Autodesk Fusion 360 part; units mm, degrees
note: some values were not read from the file. Set by a fixed rule: which sketch regions a step uses.
(part 13 of 20)
  spline S72 degree 5 poles (-2.755, -30.8773) (-2.7539, -30.8749) (-2.7515, -30.87) (-2.748, -30.8627) (-2.7434, -30.853) (-2.7376, -30.8408) (-2.7319, -30.8287) (-2.7262, -30.8165) (-2.7205, -30.8044) (-2.7149, -30.7924) (-2.7092, -30.7803) (-2.7036, -30.7683) (-2.6981, -30.7563) (-2.6925, -30.7443) (-2.687, -30.7323) (-2.6815, -30.7204) (-2.6761, -30.7085) (-2.6707, -30.6966) (-2.6653, -30.6847) (-2.6599, -30.6728) (-2.6545, -30.661) (-2.6492, -30.6492) (-2.6439, -30.6374) (-2.6387, -30.6256) (-2.6335, -30.6139) (-2.6283, -30.6022) (-2.6231, -30.5905) (-2.6179, -30.5788) (-2.6128, -30.5672) (-2.6077, -30.5555) (-2.6027, -30.5439) (-2.5977, -30.5324) (-2.5927, -30.5208) (-2.5877, -30.5093) (-2.5827, -30.4978) (-2.5778, -30.4863) (-2.5729, -30.4749) (-2.5681, -30.4634) (-2.5632, -30.452) (-2.5584, -30.4407) (-2.5537, -30.4293) (-2.5489, -30.418) (-2.5442, -30.4067) (-2.5395, -30.3954) (-2.5348, -30.3841) (-2.5302, -30.3729) (-2.5256, -30.3617) (-2.521, -30.3506) (-2.5165, -30.3394) (-2.5119, -30.3283) (-2.5074, -30.3172) (-2.503, -30.3061) (-2.4985, -30.2951) (-2.4941, -30.2841) (-2.4897, -30.2731) (-2.4854, -30.2621) (-2.481, -30.2512) (-2.4767, -30.2403) (-2.4725, -30.2294) (-2.4682, -30.2186) (-2.464, -30.2078) (-2.4598, -30.197) (-2.4557, -30.1862) (-2.4515, -30.1755) (-2.4474, -30.1648) (-2.4433, -30.1541) (-2.4393, -30.1435) (-2.4353, -30.1329) (-2.4313, -30.1223) (-2.4273, -30.1118) (-2.4234, -30.1012) (-2.4194, -30.0907) (-2.4156, -30.0803) (-2.4117, -30.0699) (-2.4079, -30.0595) (-2.4041, -30.0491) (-2.4003, -30.0388) (-2.3965, -30.0284) (-2.3928, -30.0182) (-2.3891, -30.0079) (-2.3855, -29.9977) (-2.3818, -29.9875) (-2.3782, -29.9774) (-2.3746, -29.9673) (-2.3711, -29.9572) (-2.3675, -29.9471) (-2.364, -29.9371) (-2.3606, -29.9271) (-2.3571, -29.9172) (-2.3537, -29.9073) (-2.3503, -29.8974) (-2.3469, -29.8875) (-2.3436, -29.8777) (-2.3403, -29.868) (-2.337, -29.8582) (-2.3337, -29.8485) (-2.3305, -29.8388) (-2.3273, -29.8292) (-2.3241, -29.8196) (-2.321, -29.81) (-2.3178, -29.8005) (-2.3147, -29.791) (-2.3117, -29.7815) (-2.3086, -29.7721) (-2.3056, -29.7627) (-2.3026, -29.7534) (-2.2996, -29.7441) (-2.2967, -29.7348) (-2.2938, -29.7255) (-2.2909, -29.7163) (-2.288, -29.7072) (-2.2852, -29.6981) (-2.2824, -29.689) (-2.2796, -29.6799) (-2.2769, -29.6709) (-2.2741, -29.6619) (-2.2714, -29.653) (-2.2688, -29.6441) (-2.2661, -29.6353) (-2.2635, -29.6265) (-2.2609, -29.6177) (-2.2583, -29.609) (-2.2558, -29.6003) (-2.2533, -29.5917) (-2.2508, -29.583) (-2.2483, -29.5745) (-2.2458, -29.566) (-2.2434, -29.5575) (-2.241, -29.5491) (-2.2387, -29.5407) (-2.2363, -29.5323) (-2.234, -29.524) (-2.2317, -29.5158) (-2.2295, -29.5075) (-2.2272, -29.4994) (-2.225, -29.4912) (-2.2228, -29.4832) (-2.2207, -29.4751) (-2.2185, -29.4671) (-2.2164, -29.4592) (-2.2143, -29.4513) (-2.2123, -29.4434) (-2.2102, -29.4356) (-2.2082, -29.4279) (-2.2062, -29.4202) (-2.2043, -29.4125) (-2.2023, -29.4049) (-2.2004, -29.3973) (-2.1985, -29.3898) (-2.1967, -29.3823) (-2.1948, -29.3749) (-2.193, -29.3675) (-2.1912, -29.3602) (-2.1895, -29.3529) (-2.1877, -29.3457) (-2.186, -29.3386) (-2.1843, -29.3314) (-2.1827, -29.3244) (-2.181, -29.3174) (-2.1794, -29.3104) (-2.1778, -29.3035) (-2.1762, -29.2967) (-2.1747, -29.2899) (-2.1731, -29.2831) (-2.1716, -29.2764) (-2.1702, -29.2698) (-2.1687, -29.2632) (-2.1673, -29.2567) (-2.1659, -29.2502) (-2.1645, -29.2438) (-2.1631, -29.2374) (-2.1618, -29.2311) (-2.1605, -29.2249) (-2.1592, -29.2187) (-2.1579, -29.2126) (-2.1567, -29.2065) (-2.1554, -29.2005) (-2.1542, -29.1946) (-2.153, -29.1887) (-2.1519, -29.1829) (-2.1507, -29.1771) (-2.1496, -29.1714) (-2.1485, -29.1658) (-2.1475, -29.1602) (-2.1464, -29.1547) (-2.1454, -29.1493) (-2.1444, -29.1439) (-2.1434, -29.1386) (-2.1424, -29.1334) (-2.1415, -29.1282) (-2.1406, -29.1231) (-2.1397, -29.118) (-2.1388, -29.1131) (-2.138, -29.1081) (-2.1371, -29.1033) (-2.1363, -29.0985) (-2.1355, -29.0938) (-2.1347, -29.0892) (-2.134, -29.0847) (-2.1332, -29.0802) (-2.1325, -29.0758) (-2.1318, -29.0714) (-2.1312, -29.0672) (-2.1305, -29.063) (-2.1299, -29.0589) (-2.1292, -29.0549) (-2.1286, -29.0509) (-2.1281, -29.047) (-2.1275, -29.0432) (-2.127, -29.0395) (-2.1264, -29.0359) (-2.1259, -29.0323) (-2.1254, -29.0289) (-2.125, -29.0255) (-2.1245, -29.0222) (-2.1241, -29.0189) (-2.1237, -29.0158) (-2.1233, -29.0128) (-2.1229, -29.0098) (-2.1225, -29.0069) (-2.1222, -29.0041) (-2.1219, -29.0015) (-2.1215, -28.9989) (-2.1212, -28.9963) (-2.121, -28.9939) (-2.1207, -28.9916) (-2.1204, -28.9894) (-2.1202, -28.9873) (-2.12, -28.9852) (-2.1198, -28.9833) (-2.1196, -28.9815) (-2.1194, -28.9798) (-2.1192, -28.9781) (-2.1191, -28.9766) (-2.1189, -28.9752) (-2.1188, -28.9739) (-2.1187, -28.9727) (-2.1186, -28.9716) (-2.1185, -28.9706) (-2.1184, -28.9698) (-2.1184, -28.969) (-2.1183, -28.9685) (-2.1183, -28.9682) (-2.1183, -28.968) (-2.1183, -28.9679) knots -1 -1 -1 -1 -1 -1 -0.99583333 -0.99166667 -0.9875 -0.98333333 -0.97916667 -0.975 -0.97083333 -0.96666667 -0.9625 -0.95833333 -0.95416667 -0.95 -0.94583333 -0.94166667 -0.9375 -0.93333333 -0.92916667 -0.925 -0.92083333 -0.91666667 -0.9125 -0.90833333 -0.90416667 -0.9 -0.89583333 -0.89166667 -0.8875 -0.88333333 -0.87916667 -0.875 -0.87083333 -0.86666667 -0.8625 -0.85833333 -0.85416667 -0.85 -0.84583333 -0.84166667 -0.8375 -0.83333333 -0.82916667 -0.825 -0.82083333 -0.81666667 -0.8125 -0.80833333 -0.80416667 -0.8 -0.79583333 -0.79166667 -0.7875 -0.78333333 -0.77916667 -0.775 -0.77083333 -0.76666667 -0.7625 -0.75833333 -0.75416667 -0.75 -0.74583333 -0.74166667 -0.7375 -0.73333333 -0.72916667 -0.725 -0.72083333 -0.71666667 -0.7125 -0.70833333 -0.70416667 -0.7 -0.69583333 -0.69166667 -0.6875 -0.68333333 -0.67916667 -0.675 -0.67083333 -0.66666667 -0.6625 -0.65833333 -0.65416667 -0.65 -0.64583333 -0.64166667 -0.6375 -0.63333333 -0.62916667 -0.625 -0.62083333 -0.61666667 -0.6125 -0.60833333 -0.60416667 -0.6 -0.59583333 -0.59166667 -0.5875 -0.58333333 -0.57916667 -0.575 -0.57083333 -0.56666667 -0.5625 -0.55833333 -0.55416667 -0.55 -0.54583333 -0.54166667 -0.5375 -0.53333333 -0.52916667 -0.525 -0.52083333 -0.51666667 -0.5125 -0.50833333 -0.50416667 -0.5 -0.49583333 -0.49166667 -0.4875 -0.48333333 -0.47916667 -0.475 -0.47083333 -0.46666667 -0.4625 -0.45833333 -0.45416667 -0.45 -0.44583333 -0.44166667 -0.4375 -0.43333333 -0.42916667 -0.425 -0.42083333 -0.41666667 -0.4125 -0.40833333 -0.40416667 -0.4 -0.39583333 -0.39166667 -0.3875 -0.38333333 -0.37916667 -0.375 -0.37083333 -0.36666667 -0.3625 -0.35833333 -0.35416667 -0.35 -0.34583333 -0.34166667 -0.3375 -0.33333333 -0.32916667 -0.325 -0.32083333 -0.31666667 -0.3125 -0.30833333 -0.30416667 -0.3 -0.29583333 -0.29166667 -0.2875 -0.28333333 -0.27916667 -0.275 -0.27083333 -0.26666667 -0.2625 -0.25833333 -0.25416667 -0.25 -0.24583333 -0.24166667 -0.2375 -0.23333333 -0.22916667 -0.225 -0.22083333 -0.21666667 -0.2125 -0.20833333 -0.20416667 -0.2 -0.19583333 -0.19166667 -0.1875 -0.18333333 -0.17916667 -0.175 -0.17083333 -0.16666667 -0.1625 -0.15833333 -0.15416667 -0.15 -0.14583333 -0.14166667 -0.1375 -0.13333333 -0.12916667 -0.125 -0.12083333 -0.11666667 -0.1125 -0.10833333 -0.10416667 -0.1 -0.09583333 -0.09166667 -0.0875 -0.08333333 -0.07916667 -0.075 -0.07083333 -0.06666667 -0.0625 -0.05833333 -0.05416667 -0.05 -0.04583333 -0.04166667 -0.0375 -0.03333333 -0.02916667 -0.025 -0.02083333 -0.01666667 -0.0125 -0.00833333 -0.00416667 0 0 0 0 0 0
  spline S73 degree 5 poles (26.8955, 10.9662) (26.8956, 10.9662) (26.8958, 10.9663) (26.8961, 10.9664) (26.8966, 10.9666) (26.8973, 10.9669) (26.8981, 10.9672) (26.899, 10.9676) (26.9, 10.9681) (26.9011, 10.9685) (26.9023, 10.9691) (26.9036, 10.9696) (26.905, 10.9702) (26.9065, 10.9709) (26.908, 10.9716) (26.9097, 10.9724) (26.9115, 10.9731) (26.9134, 10.974) (26.9153, 10.9749) (26.9173, 10.9758) (26.9195, 10.9768) (26.9217, 10.9778) (26.924, 10.9788) (26.9263, 10.9799) (26.9288, 10.9811) (26.9313, 10.9823) (26.9339, 10.9835) (26.9366, 10.9848) (26.9394, 10.9861) (26.9423, 10.9875) (26.9452, 10.9889) (26.9482, 10.9903) (26.9513, 10.9918) (26.9544, 10.9934) (26.9577, 10.9949) (26.961, 10.9966) (26.9643, 10.9982) (26.9678, 10.9999) (26.9713, 11.0017) (26.9748, 11.0035) (26.9785, 11.0053) (26.9822, 11.0072) (26.986, 11.0091) (26.9898, 11.0111) (26.9937, 11.0131) (26.9977, 11.0151) (27.0017, 11.0172) (27.0058, 11.0193) (27.01, 11.0215) (27.0142, 11.0237) (27.0185, 11.0259) (27.0228, 11.0282) (27.0272, 11.0306) (27.0317, 11.0329) (27.0362, 11.0353) (27.0408, 11.0378) (27.0454, 11.0403) (27.0501, 11.0428) (27.0549, 11.0454) (27.0597, 11.048) (27.0645, 11.0507) (27.0694, 11.0534) (27.0744, 11.0561) (27.0794, 11.0589) (27.0845, 11.0617) (27.0896, 11.0646) (27.0948, 11.0675) (27.1, 11.0704) (27.1053, 11.0734) (27.1106, 11.0764) (27.116, 11.0795) (27.1214, 11.0826) (27.1269, 11.0857) (27.1324, 11.0889) (27.138, 11.0921) (27.1436, 11.0954) (27.1493, 11.0987) (27.155, 11.102) (27.1608, 11.1054) (27.1666, 11.1088) (27.1725, 11.1123) (27.1784, 11.1158) (27.1843, 11.1193) (27.1903, 11.1229) (27.1963, 11.1265) (27.2024, 11.1301) (27.2085, 11.1338) (27.2147, 11.1376) (27.2209, 11.1413) (27.2271, 11.1451) (27.2334, 11.149) (27.2397, 11.1529) (27.2461, 11.1568) (27.2525, 11.1608) (27.259, 11.1648) (27.2654, 11.1688) (27.272, 11.1729) (27.2785, 11.177) (27.2851, 11.1812) (27.2918, 11.1854) (27.2985, 11.1896) (27.3052, 11.1939) (27.3119, 11.1982) (27.3187, 11.2025) (27.3256, 11.2069) (27.3324, 11.2113) (27.3393, 11.2158) (27.3463, 11.2203) (27.3533, 11.2248) (27.3603, 11.2294) (27.3673, 11.234) (27.3744, 11.2387) (27.3815, 11.2434) (27.3887, 11.2481) (27.3958, 11.2529) (27.4031, 11.2577) (27.4103, 11.2625) (27.4176, 11.2674) (27.4249, 11.2723) (27.4323, 11.2773) (27.4396, 11.2823) (27.447, 11.2873) (27.4545, 11.2924) (27.462, 11.2975) (27.4695, 11.3026) (27.477, 11.3078) (27.4846, 11.313) (27.4922, 11.3183) (27.4998, 11.3235) (27.5074, 11.3289) (27.5151, 11.3342) (27.5228, 11.3396) (27.5306, 11.3451) (27.5384, 11.3506) (27.5462, 11.3561) (27.554, 11.3616) (27.5618, 11.3672) (27.5697, 11.3728) (27.5776, 11.3785) (27.5856, 11.3842) (27.5936, 11.3899) (27.6015, 11.3957) (27.6096, 11.4015) (27.6176, 11.4074) (27.6257, 11.4132) (27.6338, 11.4192) (27.6419, 11.4251) (27.6501, 11.4311) (27.6582, 11.4371) (27.6665, 11.4432) (27.6747, 11.4493) (27.6829, 11.4554) (27.6912, 11.4616) (27.6995, 11.4678) (27.7078, 11.4741) (27.7162, 11.4803) (27.7246, 11.4867) (27.733, 11.493) (27.7414, 11.4994) (27.7498, 11.5058) (27.7583, 11.5123) (27.7668, 11.5188) (27.7753, 11.5253) (27.7838, 11.5319) (27.7924, 11.5385) (27.801, 11.5452) (27.8096, 11.5518) (27.8182, 11.5585) (27.8268, 11.5653) (27.8355, 11.5721) (27.8442, 11.5789) (27.8529, 11.5858) (27.8616, 11.5927) (27.8704, 11.5996) (27.8791, 11.6065) (27.8879, 11.6135) (27.8967, 11.6206) (27.9055, 11.6276) (27.9144, 11.6348) (27.9233, 11.6419) (27.9322, 11.6491) (27.9411, 11.6563) (27.95, 11.6635) (27.9589, 11.6708) (27.9679, 11.6781) (27.9769, 11.6855) (27.9859, 11.6929) (27.9949, 11.7003) (28.0039, 11.7078) (28.013, 11.7153) (28.0221, 11.7228) (28.0312, 11.7303) (28.0403, 11.7379) (28.0494, 11.7456) (28.0585, 11.7532) (28.0677, 11.7609) (28.0769, 11.7687) (28.0861, 11.7765) (28.0953, 11.7843) (28.1045, 11.7921) (28.1137, 11.8) (28.123, 11.8079) (28.1323, 11.8158) (28.1416, 11.8238) (28.1509, 11.8318) (28.1602, 11.8399) (28.1695, 11.848) (28.1789, 11.8561) (28.1882, 11.8643) (28.1976, 11.8724) (28.207, 11.8807) (28.2164, 11.8889) (28.2259, 11.8972) (28.2353, 11.9055) (28.2447, 11.9139) (28.2542, 11.9223) (28.2637, 11.9307) (28.2732, 11.9392) (28.2827, 11.9477) (28.2922, 11.9562) (28.3018, 11.9648) (28.3113, 11.9734) (28.3209, 11.982) (28.3305, 11.9907) (28.34, 11.9994) (28.3496, 12.0081) (28.3593, 12.0169) (28.3689, 12.0257) (28.3785, 12.0345) (28.3882, 12.0434) (28.3978, 12.0523) (28.4075, 12.0613) (28.4172, 12.0702) (28.4269, 12.0792) (28.4366, 12.0883) (28.4464, 12.0973) (28.4561, 12.1065) (28.4658, 12.1156) (28.4756, 12.1248) (28.4854, 12.134) (28.4951, 12.1432) (28.503, 12.1506) (28.5089, 12.1562) (28.5128, 12.16) (28.5147, 12.1618) knots 0 0 0 0 0 0 0.00416667 0.00833333 0.0125 0.01666667 0.02083333 0.025 0.02916667 0.03333333 0.0375 0.04166667 0.04583333 0.05 0.05416667 0.05833333 0.0625 0.06666667 0.07083333 0.075 0.07916667 0.08333333 0.0875 0.09166667 0.09583333 0.1 0.10416667 0.10833333 0.1125 0.11666667 0.12083333 0.125 0.12916667 0.13333333 0.1375 0.14166667 0.14583333 0.15 0.15416667 0.15833333 0.1625 0.16666667 0.17083333 0.175 0.17916667 0.18333333 0.1875 0.19166667 0.19583333 0.2 0.20416667 0.20833333 0.2125 0.21666667 0.22083333 0.225 0.22916667 0.23333333 0.2375 0.24166667 0.24583333 0.25 0.25416667 0.25833333 0.2625 0.26666667 0.27083333 0.275 0.27916667 0.28333333 0.2875 0.29166667 0.29583333 0.3 0.30416667 0.30833333 0.3125 0.31666667 0.32083333 0.325 0.32916667 0.33333333 0.3375 0.34166667 0.34583333 0.35 0.35416667 0.35833333 0.3625 0.36666667 0.37083333 0.375 0.37916667 0.38333333 0.3875 0.39166667 0.39583333 0.4 0.40416667 0.40833333 0.4125 0.41666667 0.42083333 0.425 0.42916667 0.43333333 0.4375 0.44166667 0.44583333 0.45 0.45416667 0.45833333 0.4625 0.46666667 0.47083333 0.475 0.47916667 0.48333333 0.4875 0.49166667 0.49583333 0.5 0.50416667 0.50833333 0.5125 0.51666667 0.52083333 0.525 0.52916667 0.53333333 0.5375 0.54166667 0.54583333 0.55 0.55416667 0.55833333 0.5625 0.56666667 0.57083333 0.575 0.57916667 0.58333333 0.5875 0.59166667 0.59583333 0.6 0.60416667 0.60833333 0.6125 0.61666667 0.62083333 0.625 0.62916667 0.63333333 0.6375 0.64166667 0.64583333 0.65 0.65416667 0.65833333 0.6625 0.66666667 0.67083333 0.675 0.67916667 0.68333333 0.6875 0.69166667 0.69583333 0.7 0.70416667 0.70833333 0.7125 0.71666667 0.72083333 0.725 0.72916667 0.73333333 0.7375 0.74166667 0.74583333 0.75 0.75416667 0.75833333 0.7625 0.76666667 0.77083333 0.775 0.77916667 0.78333333 0.7875 0.79166667 0.79583333 0.8 0.80416667 0.80833333 0.8125 0.81666667 0.82083333 0.825 0.82916667 0.83333333 0.8375 0.84166667 0.84583333 0.85 0.85416667 0.85833333 0.8625 0.86666667 0.87083333 0.875 0.87916667 0.88333333 0.8875 0.89166667 0.89583333 0.9 0.90416667 0.90833333 0.9125 0.91666667 0.92083333 0.925 0.92916667 0.93333333 0.9375 0.94166667 0.94583333 0.95 0.95416667 0.95833333 0.9625 0.96666667 0.97083333 0.975 0.97916667 0.98333333 0.9875 0.99166667 0.99583333 1 1 1 1 1 1
  line L156 (-20.11, 20.9575) -> (-20.1094, 20.9569)
  spline S74 degree 5 poles (-0.9213, -29.0307) (-0.9213, -29.0307) (-0.9213, -29.0309) (-0.9213, -29.0313) (-0.9213, -29.0318) (-0.9213, -29.0325) (-0.9213, -29.0334) (-0.9214, -29.0344) (-0.9214, -29.0355) (-0.9214, -29.0367) (-0.9214, -29.038) (-0.9214, -29.0394) (-0.9214, -29.0409) (-0.9214, -29.0425) (-0.9214, -29.0443) (-0.9214, -29.0461) (-0.9214, -29.0481) (-0.9214, -29.0501) (-0.9214, -29.0522) (-0.9214, -29.0545) (-0.9214, -29.0568) (-0.9213, -29.0592) (-0.9213, -29.0618) (-0.9212, -29.0644) (-0.9212, -29.0671) (-0.9211, -29.0699) (-0.9211, -29.0728) (-0.921, -29.0758) (-0.9209, -29.0788) (-0.9208, -29.082) (-0.9208, -29.0852) (-0.9206, -29.0886) (-0.9205, -29.092) (-0.9204, -29.0955) (-0.9203, -29.0991) (-0.9201, -29.1028) (-0.92, -29.1065) (-0.9198, -29.1103) (-0.9197, -29.1143) (-0.9195, -29.1183) (-0.9193, -29.1223) (-0.9191, -29.1265) (-0.9189, -29.1307) (-0.9186, -29.135) (-0.9184, -29.1394) (-0.9182, -29.1439) (-0.9179, -29.1484) (-0.9176, -29.153) (-0.9173, -29.1577) (-0.917, -29.1624) (-0.9167, -29.1673) (-0.9164, -29.1722) (-0.9161, -29.1771) (-0.9157, -29.1822) (-0.9153, -29.1873) (-0.915, -29.1925) (-0.9146, -29.1977) (-0.9141, -29.203) (-0.9137, -29.2084) (-0.9133, -29.2139) (-0.9128, -29.2194) (-0.9124, -29.225) (-0.9119, -29.2306) (-0.9114, -29.2363) (-0.9109, -29.2421) (-0.9103, -29.248) (-0.9098, -29.2539) (-0.9092, -29.2599) (-0.9087, -29.2659) (-0.9081, -29.272) (-0.9075, -29.2781) (-0.9068, -29.2844) (-0.9062, -29.2906) (-0.9055, -29.297) (-0.9049, -29.3034) (-0.9042, -29.3099) (-0.9035, -29.3164) (-0.9027, -29.323) (-0.902, -29.3296) (-0.9012, -29.3363) (-0.9005, -29.343) (-0.8997, -29.3498) (-0.8989, -29.3567) (-0.898, -29.3636) (-0.8972, -29.3706) (-0.8963, -29.3777) (-0.8954, -29.3847) (-0.8945, -29.3919) (-0.8936, -29.3991) (-0.8927, -29.4063) (-0.8917, -29.4137) (-0.8907, -29.421) (-0.8897, -29.4284) (-0.8887, -29.4359) (-0.8877, -29.4434) (-0.8866, -29.451) (-0.8856, -29.4586) (-0.8845, -29.4663) (-0.8834, -29.474) (-0.8822, -29.4818) (-0.8811, -29.4896) (-0.8799, -29.4975) (-0.8787, -29.5054) (-0.8775, -29.5134) (-0.8763, -29.5214) (-0.875, -29.5295) (-0.8738, -29.5376) (-0.8725, -29.5458) (-0.8712, -29.554) (-0.8698, -29.5623) (-0.8685, -29.5706) (-0.8671, -29.5789) (-0.8657, -29.5873) (-0.8643, -29.5958) (-0.8629, -29.6043) (-0.8614, -29.6128) (-0.86, -29.6214) (-0.8585, -29.6301) (-0.8569, -29.6388) (-0.8554, -29.6475) (-0.8538, -29.6563) (-0.8523, -29.6651) (-0.8507, -29.6739) (-0.849, -29.6828) (-0.8474, -29.6918) (-0.8457, -29.7008) (-0.844, -29.7098) (-0.8423, -29.7189) (-0.8406, -29.728) (-0.8388, -29.7372) (-0.8371, -29.7464) (-0.8353, -29.7556) (-0.8334, -29.7649) (-0.8316, -29.7742) (-0.8297, -29.7836) (-0.8279, -29.793) (-0.8259, -29.8025) (-0.824, -29.812) (-0.8221, -29.8215) (-0.8201, -29.8311) (-0.8181, -29.8407) (-0.8161, -29.8503) (-0.814, -29.86) (-0.812, -29.8697) (-0.8099, -29.8795) (-0.8078, -29.8893) (-0.8056, -29.8992) (-0.8035, -29.909) (-0.8013, -29.919) (-0.7991, -29.9289) (-0.7969, -29.9389) (-0.7946, -29.949) (-0.7923, -29.959) (-0.79, -29.9691) (-0.7877, -29.9793) (-0.7854, -29.9895) (-0.783, -29.9997) (-0.7806, -30.0099) (-0.7782, -30.0202) (-0.7758, -30.0306) (-0.7733, -30.0409) (-0.7708, -30.0513) (-0.7683, -30.0618) (-0.7658, -30.0722) (-0.7632, -30.0827) (-0.7606, -30.0933) (-0.758, -30.1038) (-0.7554, -30.1145) (-0.7528, -30.1251) (-0.7501, -30.1358) (-0.7474, -30.1465) (-0.7447, -30.1572) (-0.7419, -30.168) (-0.7391, -30.1788) (-0.7364, -30.1897) (-0.7335, -30.2005) (-0.7307, -30.2114) (-0.7278, -30.2224) (-0.7249, -30.2334) (-0.722, -30.2444) (-0.7191, -30.2554) (-0.7161, -30.2665) (-0.7131, -30.2776) (-0.7101, -30.2887) (-0.7071, -30.2999) (-0.704, -30.3111) (-0.7009, -30.3223) (-0.6978, -30.3336) (-0.6947, -30.3448) (-0.6915, -30.3562) (-0.6883, -30.3675) (-0.6851, -30.3789) (-0.6819, -30.3903) (-0.6786, -30.4017) (-0.6753, -30.4132) (-0.672, -30.4247) (-0.6687, -30.4362) (-0.6653, -30.4478) (-0.6619, -30.4594) (-0.6585, -30.471) (-0.6551, -30.4827) (-0.6516, -30.4943) (-0.6481, -30.506) (-0.6446, -30.5178) (-0.6411, -30.5295) (-0.6375, -30.5413) (-0.6339, -30.5531) (-0.6303, -30.565) (-0.6267, -30.5769) (-0.623, -30.5888) (-0.6193, -30.6007) (-0.6156, -30.6126) (-0.6118, -30.6246) (-0.6081, -30.6366) (-0.6043, -30.6487) (-0.6005, -30.6607) (-0.5966, -30.6728) (-0.5927, -30.685) (-0.5889, -30.6971) (-0.5849, -30.7093) (-0.581, -30.7215) (-0.577, -30.7337) (-0.573, -30.7459) (-0.569, -30.7582) (-0.5649, -30.7705) (-0.5609, -30.7828) (-0.5568, -30.7952) (-0.5526, -30.8076) (-0.5485, -30.82) (-0.5443, -30.8324) (-0.5401, -30.8448) (-0.5359, -30.8573) (-0.5316, -30.8698) (-0.5273, -30.8823) (-0.523, -30.8949) (-0.5187, -30.9075) (-0.5143, -30.9201) (-0.5099, -30.9327) (-0.5055, -30.9453) (-0.5011, -30.958) (-0.4966, -30.9707) (-0.493, -30.9809) (-0.4903, -30.9885) (-0.4885, -30.9936) (-0.4876, -30.9962) knots 0 0 0 0 0 0 0.00416667 0.00833333 0.0125 0.01666667 0.02083333 0.025 0.02916667 0.03333333 0.0375 0.04166667 0.04583333 0.05 0.05416667 0.05833333 0.0625 0.06666667 0.07083333 0.075 0.07916667 0.08333333 0.0875 0.09166667 0.09583333 0.1 0.10416667 0.10833333 0.1125 0.11666667 0.12083333 0.125 0.12916667 0.13333333 0.1375 0.14166667 0.14583333 0.15 0.15416667 0.15833333 0.1625 0.16666667 0.17083333 0.175 0.17916667 0.18333333 0.1875 0.19166667 0.19583333 0.2 0.20416667 0.20833333 0.2125 0.21666667 0.22083333 0.225 0.22916667 0.23333333 0.2375 0.24166667 0.24583333 0.25 0.25416667 0.25833333 0.2625 0.26666667 0.27083333 0.275 0.27916667 0.28333333 0.2875 0.29166667 0.29583333 0.3 0.30416667 0.30833333 0.3125 0.31666667 0.32083333 0.325 0.32916667 0.33333333 0.3375 0.34166667 0.34583333 0.35 0.35416667 0.35833333 0.3625 0.36666667 0.37083333 0.375 0.37916667 0.38333333 0.3875 0.39166667 0.39583333 0.4 0.40416667 0.40833333 0.4125 0.41666667 0.42083333 0.425 0.42916667 0.43333333 0.4375 0.44166667 0.44583333 0.45 0.45416667 0.45833333 0.4625 0.46666667 0.47083333 0.475 0.47916667 0.48333333 0.4875 0.49166667 0.49583333 0.5 0.50416667 0.50833333 0.5125 0.51666667 0.52083333 0.525 0.52916667 0.53333333 0.5375 0.54166667 0.54583333 0.55 0.55416667 0.55833333 0.5625 0.56666667 0.57083333 0.575 0.57916667 0.58333333 0.5875 0.59166667 0.59583333 0.6 0.60416667 0.60833333 0.6125 0.61666667 0.62083333 0.625 0.62916667 0.63333333 0.6375 0.64166667 0.64583333 0.65 0.65416667 0.65833333 0.6625 0.66666667 0.67083333 0.675 0.67916667 0.68333333 0.6875 0.69166667 0.69583333 0.7 0.70416667 0.70833333 0.7125 0.71666667 0.72083333 0.725 0.72916667 0.73333333 0.7375 0.74166667 0.74583333 0.75 0.75416667 0.75833333 0.7625 0.76666667 0.77083333 0.775 0.77916667 0.78333333 0.7875 0.79166667 0.79583333 0.8 0.80416667 0.80833333 0.8125 0.81666667 0.82083333 0.825 0.82916667 0.83333333 0.8375 0.84166667 0.84583333 0.85 0.85416667 0.85833333 0.8625 0.86666667 0.87083333 0.875 0.87916667 0.88333333 0.8875 0.89166667 0.89583333 0.9 0.90416667 0.90833333 0.9125 0.91666667 0.92083333 0.925 0.92916667 0.93333333 0.9375 0.94166667 0.94583333 0.95 0.95416667 0.95833333 0.9625 0.96666667 0.97083333 0.975 0.97916667 0.98333333 0.9875 0.99166667 0.99583333 1 1 1 1 1 1
  spline S75 degree 5 poles (-13.7175, 25.6019) (-13.7175, 25.602) (-13.7176, 25.6022) (-13.7178, 25.6025) (-13.718, 25.6029) (-13.7184, 25.6036) (-13.7188, 25.6043) (-13.7193, 25.6052) (-13.7198, 25.6061) (-13.7204, 25.6072) (-13.721, 25.6083) (-13.7217, 25.6096) (-13.7225, 25.6109) (-13.7233, 25.6123) (-13.7242, 25.6138) (-13.7251, 25.6154) (-13.7261, 25.6171) (-13.7271, 25.6188) (-13.7282, 25.6207) (-13.7293, 25.6226) (-13.7305, 25.6246) (-13.7317, 25.6267) (-13.733, 25.6289) (-13.7344, 25.6311) (-13.7358, 25.6334) (-13.7372, 25.6358) (-13.7387, 25.6383) (-13.7403, 25.6409) (-13.7419, 25.6435) (-13.7435, 25.6462) (-13.7452, 25.6489) (-13.747, 25.6518) (-13.7488, 25.6547) (-13.7506, 25.6577) (-13.7526, 25.6607) (-13.7545, 25.6638) (-13.7565, 25.667) (-13.7586, 25.6702) (-13.7607, 25.6735) (-13.7628, 25.6769) (-13.765, 25.6803) (-13.7673, 25.6838) (-13.7696, 25.6874) (-13.7719, 25.691) (-13.7743, 25.6947) (-13.7768, 25.6984) (-13.7793, 25.7022) (-13.7818, 25.706) (-13.7844, 25.71) (-13.787, 25.7139) (-13.7897, 25.718) (-13.7925, 25.722) (-13.7952, 25.7262) (-13.7981, 25.7304) (-13.8009, 25.7346) (-13.8039, 25.7389) (-13.8068, 25.7432) (-13.8098, 25.7476) (-13.8129, 25.7521) (-13.816, 25.7566) (-13.8192, 25.7612) (-13.8224, 25.7658) (-13.8256, 25.7704) (-13.8289, 25.7751) (-13.8322, 25.7799) (-13.8356, 25.7847) (-13.839, 25.7895) (-13.8425, 25.7944) (-13.846, 25.7993) (-13.8496, 25.8043) (-13.8532, 25.8093) (-13.8568, 25.8144) (-13.8605, 25.8195) (-13.8643, 25.8247) (-13.8681, 25.8299) (-13.8719, 25.8352) (-13.8758, 25.8405) (-13.8797, 25.8458) (-13.8836, 25.8512) (-13.8876, 25.8566) (-13.8917, 25.8621) (-13.8958, 25.8676) (-13.8999, 25.8731) (-13.9041, 25.8787) (-13.9083, 25.8843) (-13.9126, 25.89) (-13.9169, 25.8957) (-13.9213, 25.9014) (-13.9257, 25.9072) (-13.9301, 25.913) (-13.9346, 25.9188) (-13.9391, 25.9247) (-13.9437, 25.9306) (-13.9483, 25.9366) (-13.9529, 25.9426) (-13.9576, 25.9486) (-13.9624, 25.9547) (-13.9672, 25.9608) (-13.972, 25.9669) (-13.9769, 25.9731) (-13.9818, 25.9793) (-13.9867, 25.9855) (-13.9917, 25.9918) (-13.9967, 25.9981) (-14.0018, 26.0044) (-14.0069, 26.0108) (-14.0121, 26.0172) (-14.0173, 26.0236) (-14.0225, 26.0301) (-14.0278, 26.0366) (-14.0332, 26.0431) (-14.0385, 26.0497) (-14.0439, 26.0563) (-14.0494, 26.0629) (-14.0549, 26.0695) (-14.0604, 26.0762) (-14.066, 26.0829) (-14.0716, 26.0896) (-14.0772, 26.0964) (-14.0829, 26.1032) (-14.0887, 26.11) (-14.0945, 26.1168) (-14.1003, 26.1237) (-14.1061, 26.1306) (-14.112, 26.1375) (-14.118, 26.1445) (-14.1239, 26.1515) (-14.13, 26.1585) (-14.136, 26.1655) (-14.1421, 26.1726) (-14.1483, 26.1796) (-14.1544, 26.1868) (-14.1607, 26.1939) (-14.1669, 26.201) (-14.1732, 26.2082) (-14.1796, 26.2154) (-14.1859, 26.2227) (-14.1924, 26.2299) (-14.1988, 26.2372) (-14.2053, 26.2445) (-14.2119, 26.2518) (-14.2184, 26.2592) (-14.225, 26.2665) (-14.2317, 26.2739) (-14.2384, 26.2813) (-14.2451, 26.2888) (-14.2519, 26.2962) (-14.2587, 26.3037) (-14.2656, 26.3112) (-14.2724, 26.3188) (-14.2794, 26.3263) (-14.2863, 26.3339) (-14.2933, 26.3414) (-14.3004, 26.3491) (-14.3075, 26.3567) (-14.3146, 26.3643) (-14.3217, 26.372) (-14.3289, 26.3797) (-14.3362, 26.3874) (-14.3435, 26.3951) (-14.3508, 26.4029) (-14.3581, 26.4106) (-14.3655, 26.4184) (-14.3729, 26.4262) (-14.3804, 26.434) (-14.3879, 26.4419) (-14.3954, 26.4497) (-14.403, 26.4576) (-14.4106, 26.4655) (-14.4183, 26.4734) (-14.426, 26.4813) (-14.4337, 26.4893) (-14.4415, 26.4972) (-14.4493, 26.5052) (-14.4571, 26.5132) (-14.465, 26.5212) (-14.4729, 26.5292) (-14.4809, 26.5373) (-14.4889, 26.5453) (-14.4969, 26.5534) (-14.505, 26.5615) (-14.5131, 26.5696) (-14.5212, 26.5777) (-14.5294, 26.5858) (-14.5376, 26.594) (-14.5459, 26.6022) (-14.5541, 26.6103) (-14.5625, 26.6185) (-14.5708, 26.6267) (-14.5792, 26.635) (-14.5877, 26.6432) (-14.5961, 26.6514) (-14.6046, 26.6597) (-14.6132, 26.668) (-14.6218, 26.6763) (-14.6304, 26.6846) (-14.639, 26.6929) (-14.6477, 26.7012) (-14.6565, 26.7096) (-14.6652, 26.7179) (-14.674, 26.7263) (-14.6829, 26.7347) (-14.6917, 26.7431) (-14.7006, 26.7515) (-14.7096, 26.7599) (-14.7186, 26.7683) (-14.7276, 26.7767) (-14.7366, 26.7852) (-14.7457, 26.7937) (-14.7549, 26.8021) (-14.764, 26.8106) (-14.7732, 26.8191) (-14.7824, 26.8276) (-14.7917, 26.8361) (-14.801, 26.8447) (-14.8104, 26.8532) (-14.8197, 26.8618) (-14.8291, 26.8703) (-14.8386, 26.8789) (-14.8481, 26.8875) (-14.8576, 26.8961) (-14.8671, 26.9047) (-14.8767, 26.9133) (-14.8863, 26.9219) (-14.896, 26.9305) (-14.9057, 26.9392) (-14.9154, 26.9478) (-14.9252, 26.9565) (-14.935, 26.9651) (-14.9448, 26.9738) (-14.9547, 26.9825) (-14.9646, 26.9912) (-14.9745, 26.9999) (-14.9845, 27.0086) (-14.9945, 27.0173) (-15.0045, 27.026) (-15.0146, 27.0347) (-15.0247, 27.0435) (-15.0349, 27.0522) (-15.045, 27.061) (-15.0553, 27.0697) (-15.0635, 27.0767) (-15.0696, 27.082) (-15.0737, 27.0855) (-15.0758, 27.0873) knots 0 0 0 0 0 0 0.00416667 0.00833333 0.0125 0.01666667 0.02083333 0.025 0.02916667 0.03333333 0.0375 0.04166667 0.04583333 0.05 0.05416667 0.05833333 0.0625 0.06666667 0.07083333 0.075 0.07916667 0.08333333 0.0875 0.09166667 0.09583333 0.1 0.10416667 0.10833333 0.1125 0.11666667 0.12083333 0.125 0.12916667 0.13333333 0.1375 0.14166667 0.14583333 0.15 0.15416667 0.15833333 0.1625 0.16666667 0.17083333 0.175 0.17916667 0.18333333 0.1875 0.19166667 0.19583333 0.2 0.20416667 0.20833333 0.2125 0.21666667 0.22083333 0.225 0.22916667 0.23333333 0.2375 0.24166667 0.24583333 0.25 0.25416667 0.25833333 0.2625 0.26666667 0.27083333 0.275 0.27916667 0.28333333 0.2875 0.29166667 0.29583333 0.3 0.30416667 0.30833333 0.3125 0.31666667 0.32083333 0.325 0.32916667 0.33333333 0.3375 0.34166667 0.34583333 0.35 0.35416667 0.35833333 0.3625 0.36666667 0.37083333 0.375 0.37916667 0.38333333 0.3875 0.39166667 0.39583333 0.4 0.40416667 0.40833333 0.4125 0.41666667 0.42083333 0.425 0.42916667 0.43333333 0.4375 0.44166667 0.44583333 0.45 0.45416667 0.45833333 0.4625 0.46666667 0.47083333 0.475 0.47916667 0.48333333 0.4875 0.49166667 0.49583333 0.5 0.50416667 0.50833333 0.5125 0.51666667 0.52083333 0.525 0.52916667 0.53333333 0.5375 0.54166667 0.54583333 0.55 0.55416667 0.55833333 0.5625 0.56666667 0.57083333 0.575 0.57916667 0.58333333 0.5875 0.59166667 0.59583333 0.6 0.60416667 0.60833333 0.6125 0.61666667 0.62083333 0.625 0.62916667 0.63333333 0.6375 0.64166667 0.64583333 0.65 0.65416667 0.65833333 0.6625 0.66666667 0.67083333 0.675 0.67916667 0.68333333 0.6875 0.69166667 0.69583333 0.7 0.70416667 0.70833333 0.7125 0.71666667 0.72083333 0.725 0.72916667 0.73333333 0.7375 0.74166667 0.74583333 0.75 0.75416667 0.75833333 0.7625 0.76666667 0.77083333 0.775 0.77916667 0.78333333 0.7875 0.79166667 0.79583333 0.8 0.80416667 0.80833333 0.8125 0.81666667 0.82083333 0.825 0.82916667 0.83333333 0.8375 0.84166667 0.84583333 0.85 0.85416667 0.85833333 0.8625 0.86666667 0.87083333 0.875 0.87916667 0.88333333 0.8875 0.89166667 0.89583333 0.9 0.90416667 0.90833333 0.9125 0.91666667 0.92083333 0.925 0.92916667 0.93333333 0.9375 0.94166667 0.94583333 0.95 0.95416667 0.95833333 0.9625 0.96666667 0.97083333 0.975 0.97916667 0.98333333 0.9875 0.99166667 0.99583333 1 1 1 1 1 1
  arc A76 (-17.8246, 25.363) -> (-18.6136, 24.7898) centre (0, 0) ccw
  line L157 (-9.8469, 27.3243) -> (-9.7471, 27.0473)
  arc A77 (-12.5209, 25.8803) -> (-13.578, 25.3417) centre (0, 0) ccw
  arc A78 (-9.1146, 29.6298) -> (-10.0421, 29.3284) centre (0, 0) ccw
  arc A79 (-12.1618, 28.5147) -> (-13.0527, 28.1181) centre (0, 0) ccw
  spline S76 degree 5 poles (-8.0948, 27.8945) (-8.0948, 27.8946) (-8.0948, 27.8948) (-8.0949, 27.8951) (-8.0951, 27.8956) (-8.0953, 27.8963) (-8.0956, 27.8971) (-8.0958, 27.898) (-8.0962, 27.8991) (-8.0965, 27.9002) (-8.0969, 27.9015) (-8.0973, 27.9028) (-8.0978, 27.9043) (-8.0983, 27.9058) (-8.0988, 27.9075) (-8.0994, 27.9092) (-8.1, 27.9111) (-8.1007, 27.913) (-8.1013, 27.915) (-8.102, 27.9172) (-8.1028, 27.9194) (-8.1036, 27.9217) (-8.1044, 27.9241) (-8.1052, 27.9265) (-8.1061, 27.9291) (-8.107, 27.9318) (-8.108, 27.9345) (-8.109, 27.9373) (-8.11, 27.9402) (-8.1111, 27.9432) (-8.1121, 27.9462) (-8.1133, 27.9494) (-8.1144, 27.9526) (-8.1156, 27.9559) (-8.1169, 27.9593) (-8.1181, 27.9627) (-8.1194, 27.9662) (-8.1208, 27.9698) (-8.1222, 27.9735) (-8.1236, 27.9772) (-8.125, 27.9811) (-8.1265, 27.9849) (-8.128, 27.9889) (-8.1295, 27.9929) (-8.1311, 27.997) (-8.1327, 28.0012) (-8.1344, 28.0054) (-8.1361, 28.0097) (-8.1378, 28.0141) (-8.1395, 28.0185) (-8.1413, 28.023) (-8.1432, 28.0276) (-8.145, 28.0322) (-8.1469, 28.0369) (-8.1488, 28.0416) (-8.1508, 28.0464) (-8.1528, 28.0513) (-8.1548, 28.0562) (-8.1569, 28.0612) (-8.159, 28.0663) (-8.1611, 28.0714) (-8.1633, 28.0765) (-8.1655, 28.0818) (-8.1677, 28.087) (-8.17, 28.0924) (-8.1723, 28.0978) (-8.1747, 28.1032) (-8.177, 28.1087) (-8.1795, 28.1143) (-8.1819, 28.1199) (-8.1844, 28.1256) (-8.1869, 28.1313) (-8.1895, 28.1371) (-8.192, 28.1429) (-8.1947, 28.1488) (-8.1973, 28.1547) (-8.2, 28.1607) (-8.2027, 28.1667) (-8.2055, 28.1728) (-8.2083, 28.179) (-8.2111, 28.1851) (-8.214, 28.1914) (-8.2169, 28.1977) (-8.2198, 28.204) (-8.2227, 28.2104) (-8.2257, 28.2168) (-8.2288, 28.2233) (-8.2318, 28.2298) (-8.2349, 28.2363) (-8.2381, 28.2429) (-8.2412, 28.2496) (-8.2445, 28.2563) (-8.2477, 28.263) (-8.251, 28.2698) (-8.2543, 28.2767) (-8.2576, 28.2835) (-8.261, 28.2905) (-8.2644, 28.2974) (-8.2678, 28.3044) (-8.2713, 28.3115) (-8.2748, 28.3186) (-8.2784, 28.3257) (-8.282, 28.3329) (-8.2856, 28.3401) (-8.2892, 28.3473) (-8.2929, 28.3546) (-8.2966, 28.3619) (-8.3004, 28.3693) (-8.3042, 28.3767) (-8.308, 28.3842) (-8.3118, 28.3917) (-8.3157, 28.3992) (-8.3196, 28.4068) (-8.3236, 28.4144) (-8.3276, 28.422) (-8.3316, 28.4297) (-8.3357, 28.4374) (-8.3398, 28.4452) (-8.3439, 28.4529) (-8.348, 28.4608) (-8.3522, 28.4686) (-8.3565, 28.4765) (-8.3607, 28.4845) (-8.365, 28.4924) (-8.3693, 28.5004) (-8.3737, 28.5085) (-8.3781, 28.5165) (-8.3825, 28.5246) (-8.387, 28.5328) (-8.3915, 28.5409) (-8.396, 28.5491) (-8.4006, 28.5574) (-8.4052, 28.5657) (-8.4098, 28.574) (-8.4145, 28.5823) (-8.4192, 28.5907) (-8.4239, 28.5991) (-8.4287, 28.6075) (-8.4335, 28.616) (-8.4384, 28.6244) (-8.4432, 28.633) (-8.4481, 28.6415) (-8.4531, 28.6501) (-8.458, 28.6587) (-8.463, 28.6674) (-8.4681, 28.676) (-8.4732, 28.6847) (-8.4783, 28.6935) (-8.4834, 28.7022) (-8.4886, 28.711) (-8.4938, 28.7199) (-8.499, 28.7287) (-8.5043, 28.7376) (-8.5096, 28.7465) (-8.515, 28.7554) (-8.5203, 28.7644) (-8.5257, 28.7734) (-8.5312, 28.7824) (-8.5367, 28.7914) (-8.5422, 28.8005) (-8.5477, 28.8096) (-8.5533, 28.8187) (-8.5589, 28.8279) (-8.5645, 28.837) (-8.5702, 28.8462) (-8.5759, 28.8555) (-8.5817, 28.8647) (-8.5874, 28.874) (-8.5932, 28.8833) (-8.5991, 28.8926) (-8.605, 28.902) (-8.6109, 28.9113) (-8.6168, 28.9207) (-8.6228, 28.9302) (-8.6288, 28.9396) (-8.6348, 28.9491) (-8.6409, 28.9586) (-8.647, 28.9681) (-8.6532, 28.9776) (-8.6593, 28.9872) (-8.6656, 28.9968) (-8.6718, 29.0064) (-8.6781, 29.016) (-8.6844, 29.0257) (-8.6907, 29.0354) (-8.6971, 29.0451) (-8.7035, 29.0548) (-8.7099, 29.0646) (-8.7164, 29.0743) (-8.7229, 29.0841) (-8.7295, 29.0939) (-8.736, 29.1037) (-8.7426, 29.1136) (-8.7493, 29.1235) (-8.7559, 29.1334) (-8.7626, 29.1433) (-8.7694, 29.1532) (-8.7762, 29.1632) (-8.783, 29.1731) (-8.7898, 29.1831) (-8.7967, 29.1932) (-8.8036, 29.2032) (-8.8105, 29.2132) (-8.8175, 29.2233) (-8.8245, 29.2334) (-8.8315, 29.2435) (-8.8386, 29.2537) (-8.8457, 29.2638) (-8.8528, 29.274) (-8.86, 29.2842) (-8.8671, 29.2944) (-8.8744, 29.3046) (-8.8816, 29.3148) (-8.8889, 29.3251) (-8.8963, 29.3354) (-8.9036, 29.3457) (-8.911, 29.356) (-8.9184, 29.3663) (-8.9259, 29.3766) (-8.9334, 29.387) (-8.9409, 29.3974) (-8.9485, 29.4078) (-8.956, 29.4182) (-8.9637, 29.4286) (-8.9713, 29.4391) (-8.979, 29.4495) (-8.9867, 29.46) (-8.9945, 29.4705) (-9.0022, 29.481) (-9.0101, 29.4915) (-9.0179, 29.5021) (-9.0258, 29.5127) (-9.0337, 29.5232) (-9.0416, 29.5338) (-9.0496, 29.5444) (-9.0576, 29.555) (-9.0657, 29.5657) (-9.0737, 29.5763) (-9.0818, 29.587) (-9.09, 29.5977) (-9.0981, 29.6084) (-9.1047, 29.6169) (-9.1096, 29.6234) (-9.1129, 29.6276) (-9.1146, 29.6298) knots 0 0 0 0 0 0 0.00416667 0.00833333 0.0125 0.01666667 0.02083333 0.025 0.02916667 0.03333333 0.0375 0.04166667 0.04583333 0.05 0.05416667 0.05833333 0.0625 0.06666667 0.07083333 0.075 0.07916667 0.08333333 0.0875 0.09166667 0.09583333 0.1 0.10416667 0.10833333 0.1125 0.11666667 0.12083333 0.125 0.12916667 0.13333333 0.1375 0.14166667 0.14583333 0.15 0.15416667 0.15833333 0.1625 0.16666667 0.17083333 0.175 0.17916667 0.18333333 0.1875 0.19166667 0.19583333 0.2 0.20416667 0.20833333 0.2125 0.21666667 0.22083333 0.225 0.22916667 0.23333333 0.2375 0.24166667 0.24583333 0.25 0.25416667 0.25833333 0.2625 0.26666667 0.27083333 0.275 0.27916667 0.28333333 0.2875 0.29166667 0.29583333 0.3 0.30416667 0.30833333 0.3125 0.31666667 0.32083333 0.325 0.32916667 0.33333333 0.3375 0.34166667 0.34583333 0.35 0.35416667 0.35833333 0.3625 0.36666667 0.37083333 0.375 0.37916667 0.38333333 0.3875 0.39166667 0.39583333 0.4 0.40416667 0.40833333 0.4125 0.41666667 0.42083333 0.425 0.42916667 0.43333333 0.4375 0.44166667 0.44583333 0.45 0.45416667 0.45833333 0.4625 0.46666667 0.47083333 0.475 0.47916667 0.48333333 0.4875 0.49166667 0.49583333 0.5 0.50416667 0.50833333 0.5125 0.51666667 0.52083333 0.525 0.52916667 0.53333333 0.5375 0.54166667 0.54583333 0.55 0.55416667 0.55833333 0.5625 0.56666667 0.57083333 0.575 0.57916667 0.58333333 0.5875 0.59166667 0.59583333 0.6 0.60416667 0.60833333 0.6125 0.61666667 0.62083333 0.625 0.62916667 0.63333333 0.6375 0.64166667 0.64583333 0.65 0.65416667 0.65833333 0.6625 0.66666667 0.67083333 0.675 0.67916667 0.68333333 0.6875 0.69166667 0.69583333 0.7 0.70416667 0.70833333 0.7125 0.71666667 0.72083333 0.725 0.72916667 0.73333333 0.7375 0.74166667 0.74583333 0.75 0.75416667 0.75833333 0.7625 0.76666667 0.77083333 0.775 0.77916667 0.78333333 0.7875 0.79166667 0.79583333 0.8 0.80416667 0.80833333 0.8125 0.81666667 0.82083333 0.825 0.82916667 0.83333333 0.8375 0.84166667 0.84583333 0.85 0.85416667 0.85833333 0.8625 0.86666667 0.87083333 0.875 0.87916667 0.88333333 0.8875 0.89166667 0.89583333 0.9 0.90416667 0.90833333 0.9125 0.91666667 0.92083333 0.925 0.92916667 0.93333333 0.9375 0.94166667 0.94583333 0.95 0.95416667 0.95833333 0.9625 0.96666667 0.97083333 0.975 0.97916667 0.98333333 0.9875 0.99166667 0.99583333 1 1 1 1 1 1
  line L158 (-8.0945, -27.8937) -> (-8.0125, -27.6109)
  line L159 (-6.8665, -27.918) -> (-6.9368, -28.2039)
  line L160 (-10.8547, 26.6221) -> (-10.9659, 26.8948)
  spline S77 degree 5 poles (15.3132, 24.6806) (15.3132, 24.6807) (15.3133, 24.6809) (15.3135, 24.6812) (15.3138, 24.6816) (15.3142, 24.6822) (15.3146, 24.683) (15.3151, 24.6838) (15.3157, 24.6848) (15.3163, 24.6858) (15.3169, 24.6869) (15.3177, 24.6881) (15.3184, 24.6895) (15.3193, 24.6909) (15.3201, 24.6924) (15.321, 24.694) (15.322, 24.6956) (15.323, 24.6974) (15.3241, 24.6993) (15.3252, 24.7012) (15.3263, 24.7033) (15.3275, 24.7054) (15.3287, 24.7076) (15.33, 24.7099) (15.3313, 24.7122) (15.3327, 24.7147) (15.3341, 24.7172) (15.3355, 24.7198) (15.337, 24.7225) (15.3385, 24.7253) (15.34, 24.7282) (15.3416, 24.7311) (15.3432, 24.7341) (15.3449, 24.7372) (15.3465, 24.7404) (15.3482, 24.7437) (15.35, 24.747) (15.3518, 24.7504) (15.3536, 24.7539) (15.3554, 24.7574) (15.3573, 24.761) (15.3592, 24.7647) (15.3611, 24.7685) (15.3631, 24.7723) (15.3651, 24.7763) (15.3671, 24.7802) (15.3691, 24.7843) (15.3712, 24.7884) (15.3733, 24.7926) (15.3754, 24.7969) (15.3775, 24.8012) (15.3797, 24.8056) (15.3819, 24.8101) (15.3841, 24.8147) (15.3863, 24.8193) (15.3886, 24.8239) (15.3909, 24.8287) (15.3932, 24.8335) (15.3955, 24.8384) (15.3979, 24.8433) (15.4002, 24.8483) (15.4026, 24.8534) (15.405, 24.8585) (15.4075, 24.8637) (15.4099, 24.869) (15.4124, 24.8743) (15.4149, 24.8797) (15.4174, 24.8852) (15.4199, 24.8907) (15.4224, 24.8962) (15.425, 24.9019) (15.4275, 24.9076) (15.4301, 24.9133) (15.4327, 24.9192) (15.4353, 24.925) (15.438, 24.931) (15.4406, 24.937) (15.4433, 24.943) (15.446, 24.9492) (15.4486, 24.9553) (15.4514, 24.9616) (15.4541, 24.9679) (15.4568, 24.9742) (15.4595, 24.9806) (15.4623, 24.9871) (15.4651, 24.9936) (15.4678, 25.0002) (15.4706, 25.0069) (15.4734, 25.0136) (15.4762, 25.0203) (15.4791, 25.0271) (15.4819, 25.034) (15.4848, 25.0409) (15.4876, 25.0479) (15.4905, 25.0549) (15.4933, 25.062) (15.4962, 25.0691) (15.4991, 25.0763) (15.502, 25.0836) (15.5049, 25.0909) (15.5078, 25.0982) (15.5108, 25.1056) (15.5137, 25.1131) (15.5166, 25.1206) (15.5196, 25.1282) (15.5226, 25.1358) (15.5255, 25.1434) (15.5285, 25.1512) (15.5315, 25.1589) (15.5344, 25.1668) (15.5374, 25.1746) (15.5404, 25.1826) (15.5434, 25.1905) (15.5464, 25.1986) (15.5494, 25.2066) (15.5524, 25.2148) (15.5555, 25.2229) (15.5585, 25.2312) (15.5615, 25.2394) (15.5645, 25.2478) (15.5676, 25.2562) (15.5706, 25.2646) (15.5737, 25.2731) (15.5767, 25.2816) (15.5798, 25.2901) (15.5828, 25.2988) (15.5859, 25.3074) (15.5889, 25.3161) (15.592, 25.3249) (15.595, 25.3337) (15.5981, 25.3426) (15.6012, 25.3515) (15.6042, 25.3604) (15.6073, 25.3694) (15.6104, 25.3785) (15.6134, 25.3876) (15.6165, 25.3967) (15.6196, 25.4059) (15.6227, 25.4151) (15.6257, 25.4244) (15.6288, 25.4337) (15.6319, 25.4431) (15.635, 25.4525) (15.638, 25.462) (15.6411, 25.4715) (15.6442, 25.481) (15.6473, 25.4906) (15.6503, 25.5003) (15.6534, 25.5099) (15.6565, 25.5197) (15.6596, 25.5294) (15.6626, 25.5393) (15.6657, 25.5491) (15.6688, 25.559) (15.6718, 25.569) (15.6749, 25.579) (15.6779, 25.589) (15.681, 25.5991) (15.6841, 25.6092) (15.6871, 25.6194) (15.6902, 25.6296) (15.6932, 25.6398) (15.6963, 25.6501) (15.6993, 25.6604) (15.7023, 25.6708) (15.7054, 25.6812) (15.7084, 25.6917) (15.7114, 25.7022) (15.7145, 25.7127) (15.7175, 25.7233) (15.7205, 25.7339) (15.7235, 25.7446) (15.7265, 25.7553) (15.7295, 25.766) (15.7325, 25.7768) (15.7355, 25.7877) (15.7385, 25.7985) (15.7415, 25.8094) (15.7445, 25.8204) (15.7475, 25.8314) (15.7504, 25.8424) (15.7534, 25.8535) (15.7564, 25.8646) (15.7593, 25.8757) (15.7623, 25.8869) (15.7652, 25.8982) (15.7682, 25.9094) (15.7711, 25.9207) (15.774, 25.9321) (15.7769, 25.9435) (15.7798, 25.9549) (15.7828, 25.9663) (15.7857, 25.9778) (15.7886, 25.9894) (15.7914, 26.001) (15.7943, 26.0126) (15.7972, 26.0242) (15.8001, 26.0359) (15.8029, 26.0477) (15.8058, 26.0594) (15.8086, 26.0712) (15.8115, 26.0831) (15.8143, 26.095) (15.8171, 26.1069) (15.8199, 26.1188) (15.8227, 26.1308) (15.8255, 26.1428) (15.8283, 26.1549) (15.8311, 26.167) (15.8339, 26.1792) (15.8367, 26.1913) (15.8394, 26.2035) (15.8422, 26.2158) (15.8449, 26.2281) (15.8477, 26.2404) (15.8504, 26.2528) (15.8531, 26.2651) (15.8558, 26.2776) (15.8585, 26.29) (15.8612, 26.3025) (15.8639, 26.3151) (15.8666, 26.3276) (15.8692, 26.3403) (15.8719, 26.3529) (15.8745, 26.3656) (15.8771, 26.3783) (15.8798, 26.391) (15.8824, 26.4038) (15.885, 26.4166) (15.8876, 26.4295) (15.8902, 26.4424) (15.8927, 26.4553) (15.8953, 26.4682) (15.8979, 26.4812) (15.9004, 26.4943) (15.9029, 26.5073) (15.9055, 26.5204) (15.908, 26.5335) (15.9105, 26.5467) (15.913, 26.5599) (15.9154, 26.5731) (15.9174, 26.5837) (15.9189, 26.5917) (15.9199, 26.597) (15.9204, 26.5997) knots 0 0 0 0 0 0 0.00416667 0.00833333 0.0125 0.01666667 0.02083333 0.025 0.02916667 0.03333333 0.0375 0.04166667 0.04583333 0.05 0.05416667 0.05833333 0.0625 0.06666667 0.07083333 0.075 0.07916667 0.08333333 0.0875 0.09166667 0.09583333 0.1 0.10416667 0.10833333 0.1125 0.11666667 0.12083333 0.125 0.12916667 0.13333333 0.1375 0.14166667 0.14583333 0.15 0.15416667 0.15833333 0.1625 0.16666667 0.17083333 0.175 0.17916667 0.18333333 0.1875 0.19166667 0.19583333 0.2 0.20416667 0.20833333 0.2125 0.21666667 0.22083333 0.225 0.22916667 0.23333333 0.2375 0.24166667 0.24583333 0.25 0.25416667 0.25833333 0.2625 0.26666667 0.27083333 0.275 0.27916667 0.28333333 0.2875 0.29166667 0.29583333 0.3 0.30416667 0.30833333 0.3125 0.31666667 0.32083333 0.325 0.32916667 0.33333333 0.3375 0.34166667 0.34583333 0.35 0.35416667 0.35833333 0.3625 0.36666667 0.37083333 0.375 0.37916667 0.38333333 0.3875 0.39166667 0.39583333 0.4 0.40416667 0.40833333 0.4125 0.41666667 0.42083333 0.425 0.42916667 0.43333333 0.4375 0.44166667 0.44583333 0.45 0.45416667 0.45833333 0.4625 0.46666667 0.47083333 0.475 0.47916667 0.48333333 0.4875 0.49166667 0.49583333 0.5 0.50416667 0.50833333 0.5125 0.51666667 0.52083333 0.525 0.52916667 0.53333333 0.5375 0.54166667 0.54583333 0.55 0.55416667 0.55833333 0.5625 0.56666667 0.57083333 0.575 0.57916667 0.58333333 0.5875 0.59166667 0.59583333 0.6 0.60416667 0.60833333 0.6125 0.61666667 0.62083333 0.625 0.62916667 0.63333333 0.6375 0.64166667 0.64583333 0.65 0.65416667 0.65833333 0.6625 0.66666667 0.67083333 0.675 0.67916667 0.68333333 0.6875 0.69166667 0.69583333 0.7 0.70416667 0.70833333 0.7125 0.71666667 0.72083333 0.725 0.72916667 0.73333333 0.7375 0.74166667 0.74583333 0.75 0.75416667 0.75833333 0.7625 0.76666667 0.77083333 0.775 0.77916667 0.78333333 0.7875 0.79166667 0.79583333 0.8 0.80416667 0.80833333 0.8125 0.81666667 0.82083333 0.825 0.82916667 0.83333333 0.8375 0.84166667 0.84583333 0.85 0.85416667 0.85833333 0.8625 0.86666667 0.87083333 0.875 0.87916667 0.88333333 0.8875 0.89166667 0.89583333 0.9 0.90416667 0.90833333 0.9125 0.91666667 0.92083333 0.925 0.92916667 0.93333333 0.9375 0.94166667 0.94583333 0.95 0.95416667 0.95833333 0.9625 0.96666667 0.97083333 0.975 0.97916667 0.98333333 0.9875 0.99166667 0.99583333 1 1 1 1 1 1
  line L161 (-9.8472, 27.3251) -> (-9.8469, 27.3243)
  line L162 (-12.6491, 26.1453) -> (-12.5209, 25.8803)
  line L163 (12.6491, 26.1453) -> (12.6495, 26.1461)